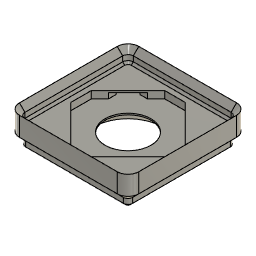
Stackable Grid Template (Autodesk Fusion 360 design; units mm, degrees)
Autodesk Fusion 360 part; units mm, degrees
sketch "Sketch1" plane through (0, 0, 0) normal (0, 0, 1) x (1, 0, 0)
  line L0 (3.75, 0) -> (37.75, 0)
  line L1 (41.5, 3.75) -> (41.5, 37.75)
  line L2 (37.75, 41.5) -> (3.75, 41.5)
  line L3 (0, 37.75) -> (0, 3.75)
  arc A0 (3.75, 41.5) -> (0, 37.75) centre (3.75, 37.75) ccw
  arc A1 (41.5, 37.75) -> (37.75, 41.5) centre (37.75, 37.75) ccw
  arc A2 (37.75, 0) -> (41.5, 3.75) centre (37.75, 3.75) ccw
  arc A3 (0, 3.75) -> (3.75, 0) centre (3.75, 3.75) ccw
  point P0 (41.5, 0)
  point P1 (0, 41.5)
  dimension "d36" = 41.5
  dimension "d37" = 41.5
  dimension "d38" = 3.75
  constraint horizontal L0
  constraint vertical L1
  constraint horizontal L2
  constraint vertical L3
  constraint coincident P1 L2
  constraint coincident P1 L3
  constraint tangent L2 A0
  constraint tangent L3 A0
  constraint tangent L1 A1
  constraint tangent L2 A1
  constraint equal A0 A1
  constraint coincident P0 L0
  constraint coincident P0 L1
  constraint tangent L0 A2
  constraint tangent L1 A2
  constraint equal A0 A2
  constraint coincident origin L0
  constraint coincident origin L3
  constraint tangent L0 A3
  constraint tangent L3 A3
  constraint equal A0 A3
  measures "d36" distance of origin P0
  measures "d37" distance of origin P1
  measures "d38" radius of A0
extrude "Extrude1" add sketch "Sketch1" along normal blind 6.4
sketch "Sketch2" plane through (0, 0, 0) normal (0, 0, -1) x (1, 0, 0)
  arc A0 (3.75, 0) -> (0, -3.75) centre (3.75, -3.75) ccw
  line L0 (0, -3.75) -> (0, -37.75)
  arc A1 (0, -37.75) -> (3.75, -41.5) centre (3.75, -37.75) ccw
  line L1 (3.75, -41.5) -> (37.75, -41.5)
  arc A2 (37.75, -41.5) -> (41.5, -37.75) centre (37.75, -37.75) ccw
  line L2 (41.5, -37.75) -> (41.5, -3.75)
  arc A3 (41.5, -3.75) -> (37.75, 0) centre (37.75, -3.75) ccw
  line L3 (37.75, 0) -> (3.75, 0)
  line L4 (3.75, 0) -> (37.75, 0)
  line L5 (41.5, -3.75) -> (41.5, -37.75)
  line L6 (37.75, -41.5) -> (3.75, -41.5)
  line L7 (0, -37.75) -> (0, -3.75)
  arc A4 (41.5, -3.75) -> (37.75, 0) centre (37.75, -3.75) ccw
  arc A5 (37.75, -41.5) -> (41.5, -37.75) centre (37.75, -37.75) ccw
  arc A6 (0, -37.75) -> (3.75, -41.5) centre (3.75, -37.75) ccw
  arc A7 (3.75, 0) -> (0, -3.75) centre (3.75, -3.75) ccw
  point P0 (41.5, 0)
  dimension "d41" = 41.5
  dimension "d42" = 3.75
  constraint horizontal L4
  constraint vertical L5
  constraint horizontal L6
  constraint vertical L7
  constraint coincident P0 L4
  constraint coincident P0 L5
  constraint tangent L4 A4
  constraint tangent L5 A4
  constraint tangent L5 A5
  constraint tangent L6 A5
  constraint equal A4 A5
  constraint tangent L6 A6
  constraint tangent L7 A6
  constraint equal A4 A6
  constraint coincident origin L4
  constraint coincident origin L7
  constraint tangent L4 A7
  constraint tangent L7 A7
  constraint equal A4 A7
  constraint equal L4 L5
  measures "d41" distance of origin P0
  measures "d42" radius of A4
extrude "Extrude2" add sketch "Sketch2" along normal blind 0.25
extrude "Extrude3" add 1 faces at (15.0833, 27.6667, -0.25) along direction (0, 0, -1) blind 2.15 draft -45
extrude "Extrude4" add 1 faces at (15.0833, 26.95, -2.4) along direction (0, 0, -1) blind 1.8
extrude "Extrude5" add 1 faces at (15.0833, 26.95, -4.2) along direction (0, 0, -1) blind 0.8 draft -45
sketch "Sketch3" plane through (0, 0, 6.4) normal (0, 0, 1) x (-1, 0, 0)
  arc A0 (0, -3.75) -> (-3.75, 0) centre (-3.75, -3.75) ccw
  line L0 (-3.75, 0) -> (-37.75, 0)
  arc A1 (-37.75, 0) -> (-41.5, -3.75) centre (-37.75, -3.75) ccw
  line L1 (-41.5, -3.75) -> (-41.5, -37.75)
  arc A2 (-41.5, -37.75) -> (-37.75, -41.5) centre (-37.75, -37.75) ccw
  line L2 (-37.75, -41.5) -> (-3.75, -41.5)
  arc A3 (-3.75, -41.5) -> (0, -37.75) centre (-3.75, -37.75) ccw
  line L3 (0, -37.75) -> (0, -3.75)
  line L4 (-3.75, 0) -> (-37.75, 0)
  line L5 (-41.5, -3.75) -> (-41.5, -37.75)
  line L6 (-37.75, -41.5) -> (-3.75, -41.5)
  line L7 (0, -37.75) -> (0, -3.75)
  arc A4 (-41.5, -37.75) -> (-37.75, -41.5) centre (-37.75, -37.75) ccw
  arc A5 (-37.75, 0) -> (-41.5, -3.75) centre (-37.75, -3.75) ccw
  arc A6 (0, -3.75) -> (-3.75, 0) centre (-3.75, -3.75) ccw
  arc A7 (-3.75, -41.5) -> (0, -37.75) centre (-3.75, -37.75) ccw
  point P0 (-41.5, 0)
  dimension "d61" = 41.5
  dimension "d62" = 3.75
  constraint horizontal L4
  constraint vertical L5
  constraint horizontal L6
  constraint vertical L7
  constraint tangent L5 A4
  constraint tangent L6 A4
  constraint coincident P0 L4
  constraint coincident P0 L5
  constraint tangent L4 A5
  constraint tangent L5 A5
  constraint equal A4 A5
  constraint coincident origin L4
  constraint coincident origin L7
  constraint tangent L4 A6
  constraint tangent L7 A6
  constraint equal A4 A6
  constraint tangent L6 A7
  constraint tangent L7 A7
  constraint equal A4 A7
  constraint equal L6 L7
  measures "d61" distance of origin P0
  measures "d62" radius of A4
extrude "Extrude6" cut sketch "Sketch3" against normal blind 1.9 draft -45
extrude "Extrude7" cut 1 faces at (26.4167, 15.7, 4.5) along direction (0, 0, -1) blind 1.8
extrude "Extrude8" cut 1 faces at (26.4167, 15.7, 2.7) along direction (0, 0, -1) blind 0.7 draft -45
sketch "Sketch4" plane through (0, 0, 2) normal (0, 0, 1) x (-1, 0, 0)
  line L0 (-2.6, -37.75) -> (-2.6, -3.75)
  arc A0 (-2.6, -3.75) -> (-3.75, -2.6) centre (-3.75, -3.75) ccw
  line L1 (-3.75, -2.6) -> (-37.75, -2.6)
  arc A1 (-37.75, -2.6) -> (-38.9, -3.75) centre (-37.75, -3.75) ccw
  line L2 (-38.9, -3.75) -> (-38.9, -37.75)
  arc A2 (-38.9, -37.75) -> (-37.75, -38.9) centre (-37.75, -37.75) ccw
  line L3 (-37.75, -38.9) -> (-3.75, -38.9)
  arc A3 (-3.75, -38.9) -> (-2.6, -37.75) centre (-3.75, -37.75) ccw
  line L4 (-7.4, -34.1) -> (-34.1, -34.1) construction
  line L5 (-34.1, -34.1) -> (-34.1, -7.4) construction
  line L6 (-34.1, -7.4) -> (-7.4, -7.4) construction
  line L7 (-7.4, -7.4) -> (-7.4, -34.1) construction
  line L8 (-20.75, -34.1) -> (-20.75, -38.9) construction
  line L9 (-34.1, -20.75) -> (-38.9, -20.75) construction
  circle A4 centre (-7.4, -34.1) radius 2.93
  circle A5 centre (-34.1, -34.1) radius 2.93
  circle A6 centre (-34.1, -7.4) radius 2.93
  circle A7 centre (-7.4, -7.4) radius 2.93
  line L10 (-4.4, -24.3118) -> (-17.1882, -37.1)
  line L11 (-17.1882, -37.1) -> (-24.3118, -37.1)
  line L12 (-24.3118, -37.1) -> (-37.1, -24.3118)
  line L13 (-37.1, -24.3118) -> (-37.1, -17.1882)
  line L14 (-37.1, -17.1882) -> (-24.3118, -4.4)
  line L15 (-24.3118, -4.4) -> (-17.1882, -4.4)
  line L16 (-17.1882, -4.4) -> (-4.4, -17.1882)
  line L17 (-4.4, -17.1882) -> (-4.4, -24.3118)
  line L18 (-4.4, -20.75) -> (-7.4, -20.75) construction
  line L19 (-20.75, -7.4) -> (-20.75, -4.4) construction
  line L20 (-9.4718, -36.1718) -> (-11.5436, -34.1)
  line L21 (-14.1882, -34.1) -> (-11.5436, -34.1)
  line L22 (-5.3282, -32.0282) -> (-7.4, -29.9564)
  line L23 (-7.4, -29.9564) -> (-7.4, -27.3118)
  line L24 (-27.3118, -34.1) -> (-29.9564, -34.1)
  line L25 (-36.1718, -32.0282) -> (-34.1, -29.9564)
  line L26 (-34.1, -29.9564) -> (-34.1, -27.3118)
  line L27 (-34.1, -14.1882) -> (-34.1, -11.5436)
  line L28 (-34.1, -11.5436) -> (-36.1718, -9.4718)
  line L29 (-27.3118, -7.4) -> (-29.9564, -7.4)
  line L30 (-29.9564, -7.4) -> (-32.0282, -5.3282)
  line L31 (-5.3282, -9.4718) -> (-7.4, -11.5436)
  line L32 (-7.4, -11.5436) -> (-7.4, -14.1882)
  line L33 (-9.4718, -5.3282) -> (-11.5436, -7.4)
  line L34 (-11.5436, -7.4) -> (-14.1882, -7.4)
  line L35 (-29.9564, -34.1) -> (-32.0282, -36.1718)
  line L36 (-2.6, -37.75) -> (-2.6, -3.75)
  arc A8 (-2.6, -3.75) -> (-3.75, -2.6) centre (-3.75, -3.75) ccw
  line L37 (-3.75, -2.6) -> (-37.75, -2.6)
  arc A9 (-37.75, -2.6) -> (-38.9, -3.75) centre (-37.75, -3.75) ccw
  line L38 (-38.9, -3.75) -> (-38.9, -37.75)
  arc A10 (-38.9, -37.75) -> (-37.75, -38.9) centre (-37.75, -37.75) ccw
  line L39 (-37.75, -38.9) -> (-3.75, -38.9)
  arc A11 (-3.75, -38.9) -> (-2.6, -37.75) centre (-3.75, -37.75) ccw
  line L40 (-2.6, -37.75) -> (-2.6, -3.75)
  arc A12 (-2.6, -3.75) -> (-3.75, -2.6) centre (-3.75, -3.75) ccw
  line L41 (-3.75, -2.6) -> (-37.75, -2.6)
  arc A13 (-37.75, -2.6) -> (-38.9, -3.75) centre (-37.75, -3.75) ccw
  line L42 (-38.9, -3.75) -> (-38.9, -37.75)
  arc A14 (-38.9, -37.75) -> (-37.75, -38.9) centre (-37.75, -37.75) ccw
  line L43 (-37.75, -38.9) -> (-3.75, -38.9)
  arc A15 (-3.75, -38.9) -> (-2.6, -37.75) centre (-3.75, -37.75) ccw
  dimension "d63" = 4.8
  dimension "d64" = 5.86
  dimension "d65" = 135
  dimension "d66" = 135
  dimension "d67" = 4.8
  dimension "d68" = 135
  dimension "d69" = 3
  dimension "d70" = 135
  dimension "d71" = 135
  constraint horizontal L4
  constraint vertical L5
  constraint horizontal L6
  constraint vertical L7
  constraint midpoint L4 L8.start
  constraint midpoint L3 L8.end
  constraint midpoint L5 L9.start
  constraint midpoint L2 L9.end
  constraint horizontal L9
  constraint vertical L8
  constraint equal L8 L9
  constraint coincident L4.start L7.end
  constraint coincident L4.end L5.start
  constraint coincident L5.end L6.start
  constraint coincident L6.end L7.start
  constraint equal A4 A5
  constraint equal A4 A6
  constraint equal A4 A7
  constraint perpendicular L9 L13
  constraint horizontal L11
  constraint horizontal L15
  constraint equal L11 L15
  constraint equal L11 L13
  constraint equal L11 L17
  constraint midpoint L17 L18.start
  constraint midpoint L7 L18.end
  constraint midpoint L6 L19.start
  constraint midpoint L15 L19.end
  constraint horizontal L18
  constraint vertical L17
  constraint vertical L19
  constraint equal L10 L12
  constraint equal L10 L14
  constraint coincident A4 L20.start
  constraint coincident L4 L20.end
  constraint tangent A4 L20
  constraint coincident L10 L21.start
  constraint coincident L4 L21.start
  constraint coincident A4 L22.start
  constraint coincident L7 L22.end
  constraint tangent A4 L22
  constraint coincident L10 L23.end
  constraint coincident L7 L23.end
  constraint coincident L4 L24.end
  constraint coincident L12 L24.start
  constraint coincident L4 L24.start
  constraint coincident A5 L25.start
  constraint tangent A5 L25
  constraint coincident L12 L26.end
  constraint coincident L5 L26.end
  constraint parallel L5 L26
  constraint coincident L5 L27.start
  constraint coincident L14 L27.start
  constraint coincident L5 L27.end
  constraint parallel L5 L27
  constraint coincident A6 L28.end
  constraint tangent A6 L28
  constraint coincident L6 L29.start
  constraint coincident L14 L29.start
  constraint coincident L6 L29.end
  constraint parallel L6 L29
  constraint coincident A6 L30.end
  constraint tangent A6 L30
  constraint coincident A7 L31.start
  constraint coincident L7 L31.end
  constraint coincident L7 L32.end
  constraint coincident L16 L32.end
  constraint coincident A7 L33.start
  constraint coincident L6 L33.end
  constraint coincident L6 L34.end
  constraint coincident L16 L34.end
  constraint coincident A5 L35.end
  constraint tangent A5 L35
  constraint tangent A7 L31
  constraint tangent A7 L33
  constraint parallel L31 L33
  constraint parallel L31 L35
  constraint parallel L25 L33
  constraint perpendicular L20 L35
  constraint parallel L20 L22
  constraint parallel L22 L30
  constraint parallel L22 L28
  measures "d63" distance of L9.start L9.end
  measures "d64" diameter of A4
  measures "d65" angle of L10 L11
  measures "d66" angle of L15 L16
  measures "d67" distance of L4.start L10
  measures "d68" angle of L12 L13
  measures "d69" distance of L19.start L19.end
  measures "d70" angle of L13 L14
  measures "d71" angle of L7 L31
extrude "Extrude9" cut sketch "Sketch4" against normal blind 2.5 contours L10 L11 L12 L13 L14 L15 L16 L17
extrude "Extrude10" cut sketch "Sketch4" against normal up to surface (1.9 mm away) from surface at -0.6 contours A4 | A4 L10 L20 L21 L22 L23 | A7 L16 L31 L32 L33 L34 | A5 L12 L24 L25 L26 L35 | A7 | A5 | A6 L14 L27 L28 L29 L30 | A6
sketch "Sketch5" plane through (0, 0, -0.5) normal (0, 0, 1) x (-1, 0, 0)
  line L0 (-14.1882, -7.4) -> (-17.1882, -4.4)
  line L1 (-17.1882, -4.4) -> (-24.3118, -4.4)
  line L2 (-24.3118, -4.4) -> (-27.3118, -7.4)
  line L3 (-27.3118, -7.4) -> (-29.9564, -7.4)
  line L4 (-29.9564, -7.4) -> (-32.0282, -5.3282)
  arc A0 (-32.0282, -5.3282) -> (-36.1718, -9.4718) centre (-34.1, -7.4) ccw
  line L5 (-36.1718, -9.4718) -> (-34.1, -11.5436)
  line L6 (-34.1, -11.5436) -> (-34.1, -14.1882)
  line L7 (-34.1, -14.1882) -> (-37.1, -17.1882)
  line L8 (-37.1, -17.1882) -> (-37.1, -24.3118)
  line L9 (-37.1, -24.3118) -> (-34.1, -27.3118)
  line L10 (-34.1, -27.3118) -> (-34.1, -29.9564)
  line L11 (-34.1, -29.9564) -> (-36.1718, -32.0282)
  arc A1 (-36.1718, -32.0282) -> (-32.0282, -36.1718) centre (-34.1, -34.1) ccw
  line L12 (-32.0282, -36.1718) -> (-29.9564, -34.1)
  line L13 (-29.9564, -34.1) -> (-27.3118, -34.1)
  line L14 (-27.3118, -34.1) -> (-24.3118, -37.1)
  line L15 (-24.3118, -37.1) -> (-17.1882, -37.1)
  line L16 (-17.1882, -37.1) -> (-14.1882, -34.1)
  line L17 (-14.1882, -34.1) -> (-11.5436, -34.1)
  line L18 (-11.5436, -34.1) -> (-9.4718, -36.1718)
  arc A2 (-9.4718, -36.1718) -> (-5.3282, -32.0282) centre (-7.4, -34.1) ccw
  line L19 (-5.3282, -32.0282) -> (-7.4, -29.9564)
  line L20 (-7.4, -29.9564) -> (-7.4, -27.3118)
  line L21 (-7.4, -27.3118) -> (-4.4, -24.3118)
  line L22 (-4.4, -24.3118) -> (-4.4, -17.1882)
  line L23 (-4.4, -17.1882) -> (-7.4, -14.1882)
  line L24 (-7.4, -14.1882) -> (-7.4, -11.5436)
  line L25 (-7.4, -11.5436) -> (-5.3282, -9.4718)
  arc A3 (-5.3282, -9.4718) -> (-9.4718, -5.3282) centre (-7.4, -7.4) ccw
  line L26 (-9.4718, -5.3282) -> (-11.5436, -7.4)
  line L27 (-11.5436, -7.4) -> (-14.1882, -7.4)
  line L28 (-20.75, -37.1) -> (-20.75, -4.4) construction
  circle A4 centre (-20.75, -20.75) radius 8
  dimension "d79" = 16
  constraint midpoint L15 L28.start
  constraint midpoint L1 L28.end
  constraint midpoint L28 A4.centre
  measures "d79" diameter of A4
extrude "Extrude12" cut sketch "Sketch5" against normal blind 0.5 contours A4
extrude "Extrude13" cut 1 faces at (25.0793, 19.3026, -1) along direction (0, 0, -1) up to surface (4 mm away) draft 45
pattern_linear "R-Pattern1" count 1 spacing 42 along (1, 0, 0) of "Extrude2", "Extrude3", "Extrude4", "Extrude5", "Extrude6", "Extrude7", "Extrude8", "Extrude9", "Extrude10", "Extrude12", "Extrude13"
equation "GridUnit = 42 mm"
equation "GridRadius = ( 8.0 / 2 ) * 1 mm"
equation "GridHeightUnit = 7 mm"
equation "GridBaseLevel1 = 0.7 mm"
equation "GridBaseLevel2 = 1.8 mm"
equation "GridBaseLevel3 = 2.15 mm"
equation "GridHeightBase = GridBaseLevel1 + GridBaseLevel2 + GridBaseLevel3"
equation "GridWidthBase = GridBaseLevel1 + GridBaseLevel3"
equation "GridGap = 0.25 mm"
equation "ProfileUnit = GridUnit - GridGap * 2"
equation "ProfileRadius = GridRadius - GridGap"
equation "ProfileBaseLevel1 = 0.8 mm"
equation "ProfileBaseLevel2 = 1.8 mm"
equation "ProfileBaseLevel3 = 2.15 mm"
equation "ProfileBaseLevel4 = GridGap"
equation "ProfileHeightBase = ProfileBaseLevel1 + ProfileBaseLevel2 + ProfileBaseLevel3 + ProfileBaseLevel4"
equation "ProfileWidthBase = ProfileBaseLevel1 + ProfileBaseLevel3"
equation "ProfileMagnetDia = 5.86 mm"
equation "ProfileMagnetOffset = 4.8 mm"
equation "ProfileMagnetDepth = 1.9 mm"
equation "ProfileLipLevel1 = 0.7 mm"
equation "ProfileLipLevel2 = 1.8 mm"
equation "ProfileLipLevel3 = 1.9 mm"
equation "ProfileHeightLip = ProfileLipLevel1 + ProfileLipLevel2 + ProfileLipLevel3"
equation "FloorOffset = 1.0 mm"
equation "Floor = GridHeightUnit - ProfileHeightBase"
equation "COLUMNS = 1"
equation "ROWS = 1"
equation "LAYERS = 0"
equation "PWidth = max(COLUMNS; 1) * GridUnit - GridGap * 2"
equation "PLength = max(ROWS; 1) * GridUnit - GridGap * 2"
equation "PHeight = max(LAYERS; 0) * GridHeightUnit + Floor"
equation "PInsideHeight = PHeight - FloorOffset"
equation "WidgetWallThickness = 2 mm"
equation "WidgetUsableWidth = PLength - WidgetWallThickness * 2"
equation "d36 = COLUMNS * GridUnit - GridGap * 2"
equation "d37 = ROWS * GridUnit - GridGap * 2"
equation "d38 = ProfileRadius"
equation "d39 = ProfileHeightLip + GridHeightUnit - ProfileHeightBase"
equation "d41 = ProfileUnit"
equation "d42 = ProfileRadius"
equation "d43 = ProfileBaseLevel4"
equation "d45 = ProfileBaseLevel3"
equation "d47 = ProfileBaseLevel2"
equation "d49 = ProfileBaseLevel1"
equation "d51 = -ProfileLipLevel3"
equation "d53 = -ProfileLipLevel2"
equation "d55 = -ProfileLipLevel1"
equation "d57 = COLUMNS"
equation "d58 = ROWS"
equation "d59 = GridUnit"
equation "d60 = GridUnit"
equation "d61 = ProfileUnit"
equation "d62 = ProfileRadius"
equation "d63 = ProfileMagnetOffset"
equation "d64 = ProfileMagnetDia"
equation "d66 = d65"
equation "d67 = ProfileMagnetOffset"
equation "d68 = d65"
equation "d70 = d65"
equation "d72 = -ProfileMagnetDepth - 0.6 mm"
